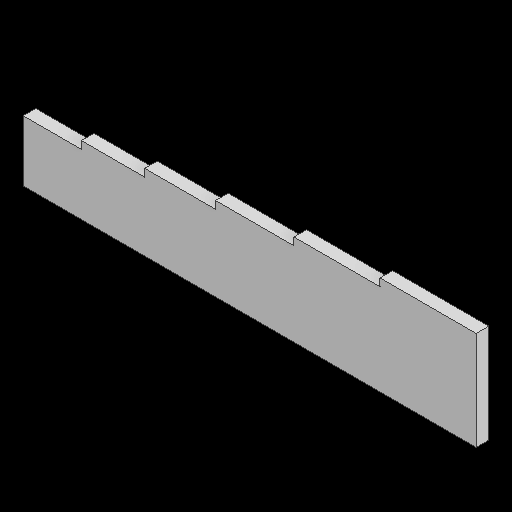
# Autodesk Inventor part: d_pocket
Saved by Autodesk Inventor 2025.1 (Build 291241000, 241)
## iProperties
Created: 2024-08-30
Part Number: d_pocket
Material: 일반
Document SubType Name: Modeling
Designer: ojs08
Density: 1 g/cm^3
Appearance: 기본값
Author: ojs08
Autodesk Inventor part; units mm, degrees
ref_plane "YZ Plane" through (0, 0, 0) normal (1, 0, 0) x (0, 1, 0)
ref_plane "XZ Plane" through (0, 0, 0) normal (0, 1, 0) x (-1, 0, 0)
ref_plane "XY Plane" through (0, 0, 0) normal (0, 0, 1) x (1, 0, 0)
sketch "스케치1" plane through (0, 0, 0) normal (0, 0, 1) x (1, 0, 0)
  line L0 (0, 0) -> (20, 0)
  line L1 (20, 0) -> (20, -20)
  line L2 (20, -20) -> (0, -20)
  line L3 (0, -20) -> (0, 0)
  line L4 (-2, 2) -> (21, 2)
  line L5 (21, 2) -> (21, -22)
  line L6 (21, -22) -> (-2, -22)
  line L7 (-2, -22) -> (-2, 2)
  line L8 (21, 2) -> (21, 5)
  line L9 (21, 5) -> (46, 5)
  line L10 (46, 5) -> (46, -22)
  line L11 (46, -22) -> (21, -22)
  line L12 (22, 3) -> (45, 3)
  line L13 (45, 3) -> (45, -20)
  line L14 (45, -20) -> (22, -20)
  line L15 (22, -20) -> (22, 3)
  line L16 (46, 5) -> (46, 8)
  line L17 (46, 8) -> (74, 8)
  line L18 (74, 8) -> (74, -22)
  line L19 (74, -22) -> (46, -22)
  line L20 (47, 6) -> (73, 6)
  line L21 (73, 6) -> (73, -20)
  line L22 (73, -20) -> (47, -20)
  line L23 (47, -20) -> (47, 6)
  line L24 (74, 8) -> (74, 11)
  line L25 (74, 11) -> (105, 11)
  line L26 (105, 11) -> (105, -22)
  line L27 (105, -22) -> (74, -22)
  line L28 (75, 9) -> (104, 9)
  line L29 (104, 9) -> (104, -20)
  line L30 (104, -20) -> (75, -20)
  line L31 (75, -20) -> (75, 9)
  line L32 (105, 11) -> (105, 14)
  line L33 (105, 14) -> (139, 14)
  line L34 (139, 14) -> (139, -22)
  line L35 (139, -22) -> (105, -22)
  line L36 (106, 12) -> (138, 12)
  line L37 (138, 12) -> (138, -20)
  line L38 (138, -20) -> (106, -20)
  line L39 (106, -20) -> (106, 12)
  line L40 (139, 14) -> (139, 17)
  line L41 (139, 17) -> (177, 17)
  line L42 (177, 17) -> (177, -22)
  line L43 (177, -22) -> (139, -22)
  line L44 (140, 15) -> (175, 15)
  line L45 (175, 15) -> (175, -20)
  line L46 (175, -20) -> (140, -20)
  line L47 (140, -20) -> (140, 15)
  dimension "d0" = 20
  dimension "d1" = 20
  dimension "d2" = 2
  dimension "d3" = 2
  dimension "d4" = 1
  dimension "d5" = 2
  dimension "d6" = 25
  dimension "d7" = 27
  dimension "d8" = 1
  dimension "d9" = 2
  dimension "d10" = 2
  dimension "d11" = 1
  dimension "d12" = 30
  dimension "d13" = 28
  dimension "d14" = 2
  dimension "d15" = 1
  dimension "d16" = 1
  dimension "d17" = 2
  dimension "d18" = 31
  dimension "d19" = 33
  dimension "d20" = 2
  dimension "d21" = 2
  dimension "d22" = 1
  dimension "d23" = 1
  dimension "d24" = 34
  dimension "d25" = 36
  dimension "d26" = 2
  dimension "d27" = 1
  dimension "d28" = 2
  dimension "d29" = 1
  dimension "d30" = 38
  dimension "d31" = 39
  dimension "d32" = 2
  dimension "d33" = 1
  dimension "d34" = 2
  dimension "d35" = 2
  constraints: 96 end point, 21 perpendicular, 14 parallel, 8 horizontal, 5 vertical, 1 coincident
  measures "d0" distance of L1.end L2.end
  measures "d1" distance of L0.end L1.end
  measures "d2" distance between parallel lines of L7 L3
  measures "d3" distance between parallel lines of L4 L0
  measures "d4" distance between parallel lines of L1 L5
  measures "d5" distance between parallel lines of L2 L6
  measures "d6" distance of L10.end L5.end
  measures "d7" distance of L9.end L10.end
  measures "d8" distance between parallel lines of L5 L15
  measures "d9" distance between parallel lines of L9 L12
  measures "d10" distance between parallel lines of L11 L14
  measures "d11" distance between parallel lines of L10 L13
  measures "d12" distance of L17.end L18.end
  measures "d13" distance of L18.end L10.end
  measures "d14" distance between parallel lines of L17 L20
  measures "d15" distance between parallel lines of L10 L23
  measures "d16" distance between parallel lines of L18 L21
  measures "d17" distance between parallel lines of L22 L19
  measures "d18" distance of L24.end L25.end
  measures "d19" distance of L25.end L26.end
  measures "d20" distance between parallel lines of L25 L28
  measures "d21" distance between parallel lines of L27 L30
  measures "d22" distance between parallel lines of L26 L29
  measures "d23" distance between parallel lines of L18 L31
  measures "d24" distance of L32.end L33.end
  measures "d25" distance of L33.end L34.end
  measures "d26" distance between parallel lines of L33 L36
  measures "d27" distance between parallel lines of L34 L37
  measures "d28" distance between parallel lines of L35 L38
  measures "d29" distance between parallel lines of L26 L39
  measures "d30" distance of L40.end L41.end
  measures "d31" distance of L41.end L42.end
  measures "d32" distance between parallel lines of L42 L45
  measures "d33" distance between parallel lines of L34 L47
  measures "d34" distance between parallel lines of L43 L46
  measures "d35" distance between parallel lines of L41 L44
extrude "돌출1" add sketch "스케치1" along normal blind 4
sketch "스케치2" plane through (0, 0, 4) normal (0, 0, 1) x (1, 0, 0)
  line L0 (-2, -22) -> (177, -22) projected
  line L1 (177, -22) -> (177, 17) projected
  line L2 (177, 17) -> (139, 17) projected
  line L3 (139, 17) -> (139, 14) projected
  line L4 (139, 14) -> (105, 14) projected
  line L5 (105, 14) -> (105, 11) projected
  line L6 (105, 11) -> (74, 11) projected
  line L7 (74, 11) -> (74, 8) projected
  line L8 (74, 8) -> (46, 8) projected
  line L9 (46, 8) -> (46, 5) projected
  line L10 (46, 5) -> (21, 5) projected
  line L11 (21, 5) -> (21, 2) projected
  line L12 (21, 2) -> (-2, 2) projected
  line L13 (-2, 2) -> (-2, -22) projected
  line L14 (22, 3) -> (45, 3) projected
  line L15 (45, 3) -> (45, -20) projected
  line L16 (45, -20) -> (22, -20) projected
  line L17 (22, -20) -> (22, 3) projected
  line L18 (47, 6) -> (73, 6) projected
  line L19 (73, 6) -> (73, -20) projected
  line L20 (73, -20) -> (47, -20) projected
  line L21 (47, -20) -> (47, 6) projected
  line L22 (75, 9) -> (104, 9) projected
  line L23 (104, 9) -> (104, -20) projected
  line L24 (104, -20) -> (75, -20) projected
  line L25 (75, -20) -> (75, 9) projected
  line L26 (106, 12) -> (138, 12) projected
  line L27 (138, 12) -> (138, -20) projected
  line L28 (138, -20) -> (106, -20) projected
  line L29 (106, -20) -> (106, 12) projected
  line L30 (140, 15) -> (175, 15) projected
  line L31 (175, 15) -> (175, -20) projected
  line L32 (175, -20) -> (140, -20) projected
  line L33 (140, -20) -> (140, 15) projected
  line L34 (0, 0) -> (20, 0) projected
  line L35 (20, 0) -> (20, -20) projected
  line L36 (20, -20) -> (0, -20) projected
  line L37 (0, -20) -> (0, 0) projected
extrude "돌출2" add sketch "스케치2" along normal blind 1 contours L13 L12 L11 L10 L9 L8 L7 L6 L5 L4 L3 L2 L1 L0 | L14 L15 L16 L17 | L18 L19 L20 L21 | L22 L23 L24 L25 | L26 L27 L28 L29 | L30 L31 L32 L33 | L34 L35 L36 L37
